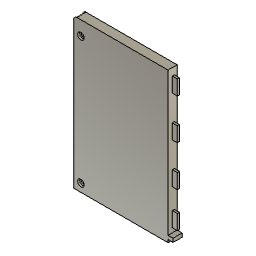
Back Plate (Autodesk Fusion 360 design; units mm, degrees)
Autodesk Fusion 360 part; units mm, degrees
sketch "Sketch1" plane through (0, 0, 0) normal (0, 1, 0) x (1, 0, 0)
  line L0 (0, 0) -> (118.11, 0)
  line L1 (118.11, 0) -> (118.11, -187.325)
  line L2 (118.11, -187.325) -> (0, -187.325)
  line L3 (0, -187.325) -> (0, 0)
  dimension "d1" = 118.11
  dimension "d2" = 187.325
  constraint horizontal L0
  constraint vertical L1
  constraint horizontal L2
  constraint vertical L3
  constraint coincident L0.start L3.end
  measures "d1" distance of L0.start L0.end
  measures "d2" distance of L0.end L1.end
extrude "Extrude1" add sketch "Sketch1" along normal blind 11.43
fillet "Fillet1" radius 3.81 1 edges at (0, 5.715, 187.325)
sketch "Sketch2" plane through (118.11, 0, 0) normal (1, 0, 0) x (0, 1, 0)
  line L0 (0, 187.325) -> (0, 0)
  line L1 (0, 0) -> (11.43, 0)
  line L2 (11.43, 0) -> (11.43, 187.325)
  line L3 (11.43, 187.325) -> (0, 187.325)
  line L4 (5.08, 178.435) -> (8.255, 178.435)
  line L5 (8.255, 178.435) -> (8.255, 159.385)
  line L6 (8.255, 159.385) -> (5.08, 159.385)
  line L7 (5.08, 159.385) -> (5.08, 178.435)
  line L8 (5.08, 127.635) -> (8.255, 127.635)
  line L9 (8.255, 127.635) -> (8.255, 108.585)
  line L10 (8.255, 108.585) -> (5.08, 108.585)
  line L11 (5.08, 108.585) -> (5.08, 127.635)
  line L12 (5.08, 76.835) -> (8.255, 76.835)
  line L13 (8.255, 76.835) -> (8.255, 57.785)
  line L14 (8.255, 57.785) -> (5.08, 57.785)
  line L15 (5.08, 57.785) -> (5.08, 76.835)
  line L16 (5.08, 32.385) -> (8.255, 32.385)
  line L17 (8.255, 32.385) -> (8.255, 13.335)
  line L18 (8.255, 13.335) -> (5.08, 13.335)
  line L19 (5.08, 13.335) -> (5.08, 32.385)
  line L20 (11.43, 8.001) -> (0, 8.001)
  line L21 (0, 8.001) -> (0, 3.429)
  line L22 (0, 3.429) -> (11.43, 3.429)
  line L23 (11.43, 3.429) -> (11.43, 8.001)
  line L24 (5.334, 32.131) -> (8.001, 32.131)
  line L25 (8.001, 32.131) -> (8.001, 13.589)
  line L26 (8.001, 13.589) -> (5.334, 13.589)
  line L27 (5.334, 13.589) -> (5.334, 32.131)
  line L28 (8.001, 76.581) -> (8.001, 58.039)
  line L29 (8.001, 58.039) -> (5.334, 58.039)
  line L30 (5.334, 58.039) -> (5.334, 76.581)
  line L31 (5.334, 76.581) -> (8.001, 76.581)
  line L32 (8.001, 127.381) -> (8.001, 108.839)
  line L33 (8.001, 108.839) -> (5.334, 108.839)
  line L34 (5.334, 108.839) -> (5.334, 127.381)
  line L35 (5.334, 127.381) -> (8.001, 127.381)
  line L36 (8.001, 178.181) -> (8.001, 159.639)
  line L37 (8.001, 159.639) -> (5.334, 159.639)
  line L38 (5.334, 159.639) -> (5.334, 178.181)
  line L39 (5.334, 178.181) -> (8.001, 178.181)
  dimension "d7" = 8.89
  dimension "d8" = 3.175
  dimension "d9" = 5.08
  dimension "d10" = 19.05
  dimension "d11" = 19.05
  dimension "d12" = 5.08
  dimension "d13" = 31.75
  dimension "d14" = 3.175
  dimension "d15" = 19.05
  dimension "d16" = 5.08
  dimension "d17" = 31.75
  dimension "d18" = 3.175
  dimension "d19" = 3.175
  dimension "d20" = 19.05
  dimension "d21" = 25.4
  dimension "d22" = 5.08
  dimension "d44" = 4.572
  dimension "d45" = 11.43
  dimension "d46" = 0.254
  dimension "d47" = 0.254
  dimension "d48" = 0.254
  dimension "d49" = 0.254
  dimension "d50" = 3.429
  constraint horizontal L4
  constraint vertical L5
  constraint horizontal L6
  constraint vertical L7
  constraint horizontal L8
  constraint vertical L9
  constraint horizontal L10
  constraint vertical L11
  constraint horizontal L12
  constraint vertical L13
  constraint horizontal L14
  constraint vertical L15
  constraint horizontal L16
  constraint vertical L17
  constraint horizontal L18
  constraint vertical L19
  constraint horizontal L20
  constraint vertical L21
  constraint horizontal L22
  constraint vertical L23
  constraint coincident L0 L21.end
  constraint collinear L0 L21
  measures "d7" distance of L3 L4
  measures "d8" distance of L4.start L4.end
  measures "d9" distance of L0 L7
  measures "d10" distance of L4.end L5.end
  measures "d11" distance of L8.end L9.end
  measures "d12" distance of L0 L11
  measures "d13" distance of L6 L8
  measures "d14" distance of L12.start L12.end
  measures "d15" distance of L12.start L14.end
  measures "d16" distance of L0 L15
  measures "d17" distance of L10 L12
  measures "d18" distance of L8.start L8.end
  measures "d19" distance of L16.start L16.end
  measures "d20" distance of L16.start L18.end
  measures "d21" distance of L14 L16
  measures "d22" distance of L0 L19
  measures "d44" distance of L20.start L22.end
  measures "d45" distance of L20.start L20.end
  measures "d50" distance of L1 L22
extrude "Extrude2" add sketch "Sketch2" along normal blind 6.35 contours L0 L2 L20 L21 L22 L23 | L24 L25 L26 L27 | L28 L29 L30 L31 | L32 L33 L34 L35 | L36 L37 L38 L39
sketch "Sketch3" plane through (0, 0, 0) normal (0, 0, -1) x (1, 0, 0)
  line L0 (118.11, 0) -> (0, 0)
  line L1 (0, 0) -> (0, -11.43)
  line L2 (0, -11.43) -> (118.11, -11.43)
  line L3 (118.11, -11.43) -> (118.11, 0)
  line L4 (6.35, -5.08) -> (25.4, -5.08)
  line L5 (25.4, -5.08) -> (25.4, -8.255)
  line L6 (25.4, -8.255) -> (6.35, -8.255)
  line L7 (6.35, -8.255) -> (6.35, -5.08)
  dimension "d25" = 19.05
  dimension "d26" = 3.175
  dimension "d27" = 6.35
  dimension "d38" = 5.08
  constraint horizontal L4
  constraint vertical L5
  constraint horizontal L6
  constraint vertical L7
  measures "d25" distance of L4.start L4.end
  measures "d26" distance of L4.start L6.end
  measures "d27" distance of L1 L7
  measures "d38" distance of L0 L4
extrude "Extrude3" add sketch "Sketch3" along normal blind 3.175 contours L4 L5 L6 L7
sketch "Sketch4" plane through (0, 0, 0) normal (0, -1, 0) x (1, 0, 0)
  arc A0 (3.81, 187.325) -> (0, 183.515) centre (3.81, 183.515) ccw
  line L0 (0, 183.515) -> (0, 0)
  line L1 (0, 0) -> (118.11, 0)
  line L2 (118.11, 0) -> (118.11, 3.429)
  line L3 (118.11, 187.325) -> (3.81, 187.325)
  line L4 (118.11, 3.429) -> (124.46, 3.429)
  line L5 (124.46, 3.429) -> (124.46, 8.001)
  line L6 (124.46, 8.001) -> (118.11, 8.001)
  line L7 (118.11, 8.001) -> (118.11, 187.325)
  point P0 (8.89, 169.545)
  point P1 (8.89, 10.16)
  dimension "d31" = 17.78
  dimension "d32" = 8.89
  dimension "d41" = 10.16
  dimension "d42" = 8.89
  measures "d31" distance of L3 P0
  measures "d32" distance of L0 P0
  measures "d41" distance of L1 P1
  measures "d42" distance of L0 P1
hole "Hole1" at (8.89, 0, 169.545) at (8.89, 0, 10.16) direction (0, 1, 0) diameter 4 depth 15.24 tip angle 180 counterbore diameter 8.255 counterbore depth 2.54
extrude "Extrude4" cut 1 faces at (12.7, 7.1967, -3.175) along direction (0, 0, 1) blind 3.175
sketch "Sketch6" plane through (0, 11.43, 0) normal (0, 1, 0) x (-1, 0, 0)
  circle A0 centre (-8.89, 169.545) radius 2
  circle A1 centre (-8.89, 10.16) radius 2
  arc A2 (0, 183.515) -> (-3.81, 187.325) centre (-3.81, 183.515) ccw
  line L0 (-3.81, 187.325) -> (-118.11, 187.325)
  line L1 (-118.11, 187.325) -> (-118.11, 8.001)
  line L2 (-118.11, 8.001) -> (-124.46, 8.001)
  line L3 (-124.46, 8.001) -> (-124.46, 3.429)
  line L4 (-124.46, 3.429) -> (-118.11, 3.429)
  line L5 (-118.11, 3.429) -> (-118.11, 0)
  line L6 (-118.11, 0) -> (0, 0)
  line L7 (0, 0) -> (0, 183.515)
  line L8 (-86.36, 0) -> (-35.56, 0)
  line L9 (-35.56, 0) -> (-35.56, 50.8)
  line L10 (-35.56, 50.8) -> (-86.36, 50.8)
  line L11 (-86.36, 50.8) -> (-86.36, 0)
  point P0 (-60.96, 187.325)
  point P1 (-60.96, 50.8)
  dimension "d51" = 50.8
  dimension "d52" = 50.8
  constraint horizontal L8
  constraint vertical L9
  constraint horizontal L10
  constraint vertical L11
  constraint coincident L6 L8.start
  constraint midpoint L0 P0
  constraint midpoint L10 P1
  constraint vertical P0 P1
  constraint collinear L6 L8
  measures "d51" distance of L9.end L10.end
  measures "d52" distance of L8.end L9.end
extrude "Extrude5" cut sketch "Sketch6" against normal blind 5.08 contours L6 L8 L9 L10 L11
